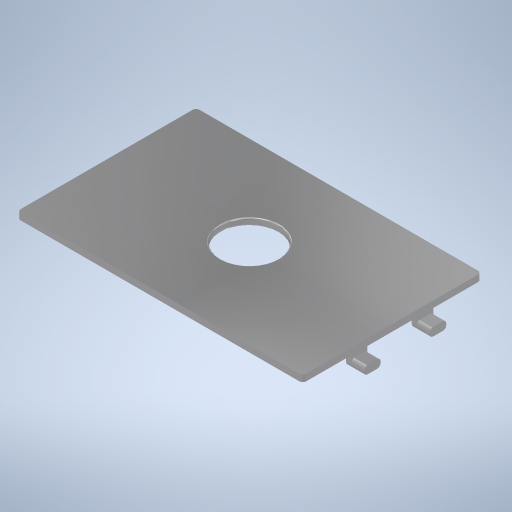
# Autodesk Inventor part: tapa de caja
Saved by Autodesk Inventor 2023 (Build 270158000, 158)
## iProperties
Created: 2022-11-16
Part Number: tapa de caja
Material: Generic
Document SubType Name: Modeling
Designer: Xiaba
Density: 1 g/cm^3
Appearance: Default
Author: Xiaba
Autodesk Inventor part; units mm, degrees
ref_plane "YZ Plane" through (0, 0, 0) normal (1, 0, 0) x (0, 1, 0)
ref_plane "XZ Plane" through (0, 0, 0) normal (0, 1, 0) x (-1, 0, 0)
ref_plane "XY Plane" through (0, 0, 0) normal (0, 0, 1) x (1, 0, 0)
sketch "Sketch1" plane through (0, 0, 0) normal (0, 1, 0) x (-1, 0, 0)
  line L0 (86.9, 54.4) -> (-86.9, 54.4)
  line L1 (-86.9, 54.4) -> (-86.9, -54.4)
  line L2 (-86.9, -54.4) -> (86.9, -54.4)
  line L3 (86.9, -54.4) -> (86.9, 54.4)
  line L4 (86.9, 54.4) -> (-86.9, -54.4) construction
  line L5 (-86.9, 54.4) -> (86.9, -54.4) construction
  point P0 (0, 0)
  dimension "d0" = 108.8
  dimension "d1" = 173.8
  constraints: 12 end point, 2 midpoint, 2 parallel, 1 horizontal, 1 perpendicular
  measures "d0" distance of L2.end L0.start
  measures "d1" distance of L1.end L2.end
extrude "Extrusion1" add sketch "Sketch1" along normal blind 4
sketch "Sketch2" plane through (86.9, 0, 54.4) normal (1, 0, 0) x (0, 0, -1)
  line L0 (39.4, 6.5316) -> (69.4, 6.5316)
  line L1 (69.4, 6.5316) -> (69.4, -6.5316)
  line L2 (69.4, -6.5316) -> (39.4, -6.5316)
  line L3 (39.4, -6.5316) -> (39.4, 6.5316)
  line L4 (39.4, 6.5316) -> (69.4, -6.5316) construction
  line L5 (69.4, 6.5316) -> (39.4, -6.5316) construction
  line L6 (69.4, 0) -> (79.4, 0)
  line L7 (79.4, 0) -> (79.4, -2)
  line L8 (79.4, -2) -> (69.4, -2)
  line L9 (69.4, -2) -> (69.4, 0)
  line L10 (39.4, 0) -> (29.4, 0)
  line L11 (29.4, 0) -> (29.4, -2)
  line L12 (29.4, -2) -> (39.4, -2)
  line L13 (39.4, -2) -> (39.4, 0)
  line L14 (69.4, -2) -> (79.4, -2)
  line L15 (79.4, -2) -> (79.4, -7)
  line L16 (79.4, -7) -> (69.4, -7)
  line L17 (69.4, -7) -> (69.4, -2)
  line L18 (39.4, -2) -> (29.4, -2)
  line L19 (29.4, -2) -> (29.4, -7)
  line L20 (29.4, -7) -> (39.4, -7)
  line L21 (39.4, -7) -> (39.4, -2)
  point P0 (54.4, 0)
  point P1 (69.4, -6.5316)
  dimension "d4" = 30
  dimension "d5" = 2
  dimension "d6" = 2
  dimension "d7" = 5
  dimension "d8" = 10
  dimension "d9" = 5
  dimension "d10" = 10
  dimension "d11" = 10
  dimension "d12" = 10
  constraints: 44 end point, 10 parallel, 5 horizontal, 5 perpendicular, 4 midpoint
  measures "d4" distance of L0.start L0.end
  measures "d5" distance of L10.end L11.end
  measures "d6" distance of L6.end L7.end
  measures "d7" distance of L18.end L19.end
  measures "d8" distance of L19.end L20.end
  measures "d9" distance of L14.end L15.end
  measures "d10" distance of L15.end L16.end
  measures "d11" distance of L6.start L6.end
  measures "d12" distance of L10.start L10.end
extrude "Extrusion2" add sketch "Sketch2" against normal blind 3 contours L3 L12 L11 L10 | L6 L7 L8 L1 | L3 L21 L20 L19 L12 | L8 L15 L16 L17 L1
sketch "Sketch3" plane through (86.9, 0, -54.4) normal (1, 0, 0) x (0, 0, -1)
  line L0 (-79.4, -2) -> (-69.4, -2) projected
  line L1 (-69.4, -7) -> (-69.4, -2) projected
  line L2 (-79.4, -7) -> (-69.4, -7) projected
  line L3 (-79.4, -2) -> (-79.4, -7) projected
  line L4 (-29.4, -2) -> (-39.4, -2) projected
  line L5 (-29.4, -2) -> (-29.4, -7) projected
  line L6 (-29.4, -7) -> (-39.4, -7) projected
  line L7 (-39.4, -7) -> (-39.4, -2) projected
  line L8 (-79.4, -7) -> (-69.4, -7) projected
  line L9 (-77.4, -2) -> (-71.4, -2)
  line L10 (-69.4, -4) -> (-69.4, -5)
  line L11 (-71.4, -7) -> (-77.4, -7)
  line L12 (-79.4, -5) -> (-79.4, -4)
  line L13 (-37.4, -2) -> (-31.4, -2)
  line L14 (-29.4, -4) -> (-29.4, -5)
  line L15 (-31.4, -7) -> (-37.4, -7)
  line L16 (-39.4, -5) -> (-39.4, -4)
  arc A0 (-37.4, -2) -> (-39.4, -4) centre (-37.4, -4) ccw
  arc A1 (-29.4, -4) -> (-31.4, -2) centre (-31.4, -4) ccw
  arc A2 (-31.4, -7) -> (-29.4, -5) centre (-31.4, -5) ccw
  arc A3 (-39.4, -5) -> (-37.4, -7) centre (-37.4, -5) ccw
  arc A4 (-77.4, -2) -> (-79.4, -4) centre (-77.4, -4) ccw
  arc A5 (-69.4, -4) -> (-71.4, -2) centre (-71.4, -4) ccw
  arc A6 (-71.4, -7) -> (-69.4, -5) centre (-71.4, -5) ccw
  arc A7 (-79.4, -5) -> (-77.4, -7) centre (-77.4, -5) ccw
  point P0 (-54.4, 0)
  dimension "d15" = 2
  constraints: 16 end point, 16 point on circle, 16 tangent, 8 centre point, 8 point on line, 7 equal radius, 4 parallel, 2 horizontal, 2 perpendicular
  measures "d15" radius of A0
extrude "Extrusion3" add sketch "Sketch3" along normal blind 8 contours L0 A5 L1 A6 L2 A7 L3 A4 | A1 L5 A2 L6 A3 L7 A0 L4
sketch "Sketch4" plane through (94.9, 0, -54.4) normal (1, 0, 0) x (0, 0, -1)
  line L0 (-77.4, -7) -> (-71.4, -7) projected
  arc A0 (-71.4, -7) -> (-69.4, -5) centre (-71.4, -5) ccw projected
  line L1 (-69.4, -5) -> (-69.4, -4) projected
  arc A1 (-69.4, -4) -> (-71.4, -2) centre (-71.4, -4) ccw projected
  line L2 (-71.4, -2) -> (-77.4, -2) projected
  arc A2 (-77.4, -2) -> (-79.4, -4) centre (-77.4, -4) ccw projected
  line L3 (-79.4, -4) -> (-79.4, -5) projected
  arc A3 (-79.4, -5) -> (-77.4, -7) centre (-77.4, -5) ccw projected
  line L4 (-37.4, -7) -> (-31.4, -7) projected
  arc A4 (-31.4, -7) -> (-29.4, -5) centre (-31.4, -5) ccw projected
  line L5 (-29.4, -5) -> (-29.4, -4) projected
  arc A5 (-29.4, -4) -> (-31.4, -2) centre (-31.4, -4) ccw projected
  line L6 (-31.4, -2) -> (-37.4, -2) projected
  arc A6 (-37.4, -2) -> (-39.4, -4) centre (-37.4, -4) ccw projected
  line L7 (-39.4, -4) -> (-39.4, -5) projected
  arc A7 (-39.4, -5) -> (-37.4, -7) centre (-37.4, -5) ccw projected
  line L8 (-79.4, 0) -> (-79.4, -4) projected
  line L9 (-79.4, -2) -> (-69.4, -2)
  line L10 (-69.4, -2) -> (-69.4, -8.3081)
  line L11 (-69.4, -8.3081) -> (-79.4, -8.3081)
  line L12 (-79.4, -8.3081) -> (-79.4, -2)
  line L13 (-39.4, -7) -> (-39.4, 0) projected
  line L14 (-39.4, -2) -> (-29.4, -2)
  line L15 (-29.4, -2) -> (-29.4, -9.9458)
  line L16 (-29.4, -9.9458) -> (-39.4, -9.9458)
  line L17 (-39.4, -9.9458) -> (-39.4, -2)
  point P0 (-54.4, 0)
  point P1 (-29.4, -5)
  constraints: 16 end point, 4 parallel, 2 horizontal, 2 perpendicular, 2 point on line, 1 midpoint
extrude "Extrusion4" cut sketch "Sketch4" against normal through all contours L0 A0 L10 L11 L12 A3 | L4 A4 L15 L16 L17 L13 A7
fillet "Fillet1" radius 2 4 edges at (86.9, 2, 54.4) (86.9, 2, -54.4) (-86.9, 2, -54.4) (-86.9, 2, 54.4)
sketch "Sketch5" plane through (0, 4, 0) normal (0, 1, 0) x (1, 0, 0)
  circle A0 centre (0, 0) radius 17.5
  dimension "d21" = 35
  constraints: 1 centre point, 1 coincident
  measures "d21" diameter of A0
extrude "Extrusion5" cut sketch "Sketch5" against normal blind 10
fillet "Fillet2" radius 1 2 edges at (-17.5, 0, 0) (-17.5, 4, 0)
body "Solid1"
